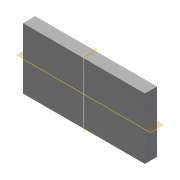
# Autodesk Inventor part: Part1
Saved by Autodesk Inventor 2022 (Build 260148000, 148)
## iProperties
Created: 2006-01-12
Part Number: Part1
Document SubType Name: Modeling
Designer: Administrator
Material: Steel, Mild
Density: 7.86 g/cm^3
Appearance: Steel
Author: Administrator
Autodesk Inventor part; units mm, degrees
ref_plane "XY Plane" through (0, 0, 0) normal (0, 0, 1) x (1, 0, 0)
sketch "Sketch1" plane through (0, 0, 0) normal (0, 0, 1) x (1, 0, 0)
  line L0 (-127, 63.5) -> (127, 63.5)
  line L1 (127, 63.5) -> (127, -63.5)
  line L2 (127, -63.5) -> (-127, -63.5)
  line L3 (-127, -63.5) -> (-127, 63.5)
  line L4 (0, 88.9) -> (0, -88.9) projected
  line L5 (-177.8, 0) -> (177.8, 0) projected
  dimension "d0" = 254
  dimension "d1" = 127
  constraints: 8 end point, 2 parallel, 1 horizontal, 1 perpendicular, 2 other
  measures "d0" distance of L0.start L0.end
  measures "d1" distance of L2.end L0.start
extrude "Extrusion1" add sketch "Sketch1" along normal blind 25.4
body "Solid1"
